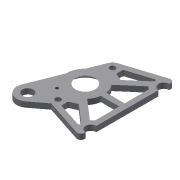
# Autodesk Inventor part: v2_tri_headplate_parameter_REF
Saved by Autodesk Inventor 2019 (Build 230136000, 136)
## iProperties
Created: 2017-06-27
Part Number: v2_tri_headplate_parameter_REF
Material: Generic
Document SubType Name: Modeling
Designer: richp
Density: 1 g/cm^3
Appearance: Default
headplate_aperture_diameter: 0.450 in
headplate_thickness: 0.124 in
ball_bearing_radius: 0.125 in
Author: richp
Autodesk Inventor part; units mm, degrees
sketch "Sketch1" plane through (0, 0, 0) normal (0, 1, 0) x (-1, 0, 0)
  circle A0 centre (0, 0) radius 5.715
  circle A1 centre (0, 0) radius 24.4983 construction
  line L0 (38.3553, 0) -> (-43.5095, 0) construction
  line L1 (0, -41.4931) -> (0, 53.8329) construction
  line L2 (-24.4983, 0) -> (-24.4983, -14.859)
  arc A2 (-24.4983, -24.384) -> (-24.4983, -18.034) centre (-24.4983, -21.209) ccw
  arc A3 (-24.4983, 24.384) -> (-24.4983, 18.034) centre (-24.4983, 21.209) ccw construction
  line L3 (-24.4983, 21.209) -> (-24.4983, 18.034) construction
  arc A4 (-24.4983, 14.859) -> (-21.3233, 15.7097) centre (-24.4983, 21.209) ccw construction
  arc A5 (-21.9753, -27.0363) -> (-20.631, -26.2455) centre (-24.4983, -21.209) ccw construction
  line L4 (-24.4983, 14.859) -> (-24.4983, 0)
  line L5 (-24.4983, -14.859) -> (-24.4983, -18.034)
  arc A6 (-22.4188, -15.2092) -> (-24.4983, -27.559) centre (-24.4983, -21.209) ccw construction
  arc A7 (-24.4983, -18.034) -> (-24.4983, -24.384) centre (-24.4983, -21.209) ccw construction
  line L6 (-24.4983, 21.209) -> (-24.4983, 24.384) construction
  arc A8 (-24.4983, 18.034) -> (-24.4983, 24.384) centre (-24.4983, 21.209) ccw
  line L7 (-24.4983, 24.384) -> (-24.4983, 25.0867)
  line L8 (-24.4983, -24.384) -> (-24.4983, -25.0929)
  line L9 (-24.4983, 18.034) -> (-24.4983, 14.859)
  line L10 (-24.4983, -18.034) -> (-24.4983, -24.384) construction
  line L11 (0, 0) -> (-8.1614, 7.0656) construction
  line L12 (0, 0) -> (-8.1614, -7.0656) construction
  line L13 (0, 0) -> (24.493, 0) construction
  arc A9 (9.9646, -4.1519) -> (9.9646, 4.1519) centre (0, 0) ccw construction
  line L14 (-5.7223, -9.1535) -> (-5.719, -9.1507) construction
  line L15 (-9.8786, -4.3527) -> (-22.4188, -15.2092) construction
  line L16 (-21.3233, 15.7097) -> (-21.3233, -15.7097)
  arc A10 (7.4735, -7.7897) -> (9.7402, -4.654) centre (0, 0) ccw construction
  line L17 (-5.719, -9.1507) -> (-18.2625, -20.01) construction
  arc A11 (-18.1902, -21.9377) -> (-18.2625, -20.01) centre (-24.4983, -21.209) ccw construction
  arc A12 (-18.2625, -20.01) -> (-19.6975, -17.0527) centre (-24.4983, -21.209) ccw construction
  line L18 (-8.1614, -7.0656) -> (-19.6975, -17.0527)
  arc A13 (-19.6975, -17.0527) -> (-21.3233, -15.7097) centre (-24.4983, -21.209) ccw
  arc A14 (-8.1614, 7.0656) -> (-8.1614, -7.0656) centre (0, 0) ccw
  line L19 (-19.6975, 17.0527) -> (-24.4983, 21.209) construction
  arc A15 (-21.3233, 15.7097) -> (-19.6975, 17.0527) centre (-24.4983, 21.209) ccw
  arc A16 (-21.3233, -15.7097) -> (-22.4188, -15.2092) centre (-24.4983, -21.209) ccw construction
  line L20 (-8.1614, 7.0656) -> (-18.5216, 16.0348)
  arc A17 (-8.1614, -7.0656) -> (6.5744, -8.562) centre (0, 0) ccw construction
  line L21 (-8.1614, -7.0656) -> (-19.6975, -17.0527) construction
  arc A18 (-21.3233, -15.7097) -> (-24.4983, -14.859) centre (-24.4983, -21.209) ccw construction
  line L22 (-19.6975, -17.0527) -> (-24.4983, -21.209) construction
  arc A19 (-19.6975, -17.0527) -> (-21.3233, -15.7097) centre (-24.4983, -21.209) ccw construction
  line L23 (-18.5216, 16.0348) -> (-19.6975, 17.0527)
  arc A20 (-19.6975, 17.0527) -> (-18.7927, 23.9963) centre (-24.4983, 21.209) ccw construction
  arc A21 (9.9646, 4.1519) -> (8.0122, 7.2344) centre (0, 0) ccw construction
  arc A22 (7.4735, 7.7897) -> (5.3975, 9.3487) centre (0, 0) ccw construction
  line L24 (0, 0) -> (5.3975, 9.3487) construction
  circle A23 centre (12.2491, 21.2162) radius 3.175
  arc A24 (15.4241, 26.7154) -> (12.0688, 27.5636) centre (12.2491, 21.2162) ccw
  arc A25 (17.9787, 18.4785) -> (18.1476, 18.8644) centre (12.2491, 21.2162) ccw construction
  arc A26 (12.0688, 27.5636) -> (8.7197, 26.4949) centre (12.2491, 21.2162) ccw
  arc A27 (-24.4983, -27.559) -> (-22.566, -27.2579) centre (-24.4983, -21.209) ccw construction
  arc A28 (-20.631, -26.2455) -> (-18.1902, -21.9377) centre (-24.4983, -21.209) ccw construction
  arc A29 (-20.631, -26.2455) -> (-19.6975, -17.0527) centre (-24.4983, -21.209) ccw construction
  arc A30 (6.5744, -8.562) -> (7.4735, -7.7897) centre (0, 0) ccw construction
  arc A31 (9.7402, -4.654) -> (9.9646, -4.1519) centre (0, 0) ccw construction
  arc A32 (6.7499, 18.0412) -> (7.1395, 17.446) centre (12.2491, 21.2162) ccw construction
  arc A33 (6.7484, 24.3886) -> (6.7499, 18.0412) centre (12.2491, 21.2162) ccw construction
  arc A34 (-0.7648, 10.7679) -> (-8.1614, 7.0656) centre (0, 0) ccw construction
  arc A35 (-18.7927, 23.9963) -> (-18.999, 24.384) centre (-24.4983, 21.209) ccw construction
  arc A36 (-18.999, 24.384) -> (-21.9753, 27.0363) centre (-24.4983, 21.209) ccw construction
  arc A37 (-21.9753, 27.0363) -> (-22.5177, 27.2422) centre (-24.4983, 21.209) ccw construction
  arc A38 (-24.4987, 27.559) -> (-24.4983, 14.859) centre (-24.4983, 21.209) ccw construction
  arc A39 (0, -11.8491) -> (3.716, -17.3312) centre (0, -15.8496) ccw construction
  circle A40 centre (0, 15.8496) radius 4.0005 construction
  line L25 (3.0165, -19.0856) -> (3.716, -17.3312) construction
  arc A41 (18.1476, 18.8644) -> (15.4241, 26.7154) centre (12.2491, 21.2162) ccw
  line L26 (3.0165, -19.0856) -> (1.2173, -19.6604) construction
  arc A42 (9.0741, 15.7169) -> (11.5389, 14.906) centre (12.2491, 21.2162) ccw construction
  arc A43 (5.3975, 9.3487) -> (2.2591, 10.556) centre (0, 0) ccw construction
  line L27 (9.0741, 15.7169) -> (22.677, 39.2777) construction
  line L28 (5.3975, 9.3487) -> (9.0741, 15.7169) construction
  arc A44 (11.5389, 14.906) -> (17.9787, 18.4785) centre (12.2491, 21.2162) ccw construction
  arc A45 (7.1395, 17.446) -> (9.0741, 15.7169) centre (12.2491, 21.2162) ccw construction
  arc A46 (2.2591, 10.556) -> (1.3866, 10.7056) centre (0, 0) ccw construction
  arc A47 (8.0122, 7.2344) -> (7.4735, 7.7897) centre (0, 0) ccw construction
  arc A48 (8.7197, 26.4949) -> (18.1476, 18.8644) centre (12.2491, 21.2162) ccw construction
  arc A49 (-22.5656, 27.2577) -> (-24.4983, 27.559) centre (-24.4983, 21.209) ccw construction
  arc A50 (-22.566, -27.2579) -> (-20.631, -26.2455) centre (-24.4983, -21.209) ccw construction
  arc A51 (3.716, -17.3312) -> (0, -11.8491) centre (0, -15.8496) ccw construction
  line L29 (0, -20.0493) -> (-21.848, -27.0285)
  arc A52 (1.2173, -19.6604) -> (3.716, -17.3312) centre (0, -15.8496) ccw
  line L30 (0, 19.8501) -> (-21.8325, 27.0173)
  arc A53 (-22.5177, 27.2422) -> (-22.5656, 27.2577) centre (-24.4983, 21.209) ccw construction
  line L31 (0, 19.8501) -> (8.3945, 26.2624)
  arc A54 (8.3945, 26.2624) -> (6.7484, 24.3886) centre (12.2491, 21.2162) ccw construction
  arc A55 (-21.8325, 27.0173) -> (-24.4983, 25.0867) centre (-22.4663, 25.0867) ccw
  arc A56 (-24.4983, -25.0929) -> (-21.848, -27.0285) centre (-22.4663, -25.0929) ccw
  line L32 (-21.8325, 27.0173) -> (-24.4983, 27.8924) construction
  line L33 (-24.4983, 24.384) -> (-24.4983, 27.8924) construction
  line L34 (-21.848, -27.0285) -> (-24.4983, -27.8751) construction
  line L35 (-24.4983, -25.0929) -> (-24.4983, -27.8751) construction
  line L36 (8.3945, 26.2624) -> (26.6603, 40.2149) construction
  line L37 (18.1476, 18.8644) -> (26.6603, 40.2149) construction
  line L38 (1.2173, -19.6604) -> (0, -20.0493)
  line L39 (3.716, -17.3312) -> (18.1476, 18.8644)
  arc A57 (18.1476, 18.8644) -> (8.3945, 26.2624) centre (12.2491, 21.2162) ccw
  dimension "headplate_aperture_diameter" = 11.43
  dimension "mount_diameter" = 48.9966
  dimension "d3" = 6.35
  dimension "d4" = 42.418
  dimension "d5" = 31.6992
  dimension "d7" = 3.175
  dimension "d8" = 3.175
  dimension "d10" = 5.08
  dimension "d11" = 3.175
  dimension "d12" = 3.175
  dimension "d16" = 3.175
  dimension "d33" = 120
  dimension "d34" = 6.35
  dimension "d36" = 3.175
  dimension "d46" = 8.001
  dimension "d75" = 2.032
  constraints: 143 point on circle, 76 end point, 57 centre point, 26 tangent, 16 point on line, 11 collinear, 10 vertical, 6 coincident, 4 symmetric about line, 3 parallel, 1 equal radius, 1 horizontal, 1 midpoint, 1 vertical alignment, 5 other
  measures "headplate_aperture_diameter" diameter of A0
  measures "mount_diameter" diameter of A1
  measures "d3" diameter of A2
  measures "d4" distance of L3.start A2.centre
  measures "d5" distance of point (0, -15.85) point (0, 15.85)
  measures "d7" radial gap between concentric circles of A3 A4
  measures "d8" radial gap between concentric circles of A2 A5
  measures "d10" radial gap between concentric circles of A0 A9
  measures "d11" distance between parallel lines of L12 L14
  measures "d12" distance between parallel lines of L12 L15
  measures "d16" distance between parallel lines of L4 L16
  measures "d33" angle of L0 L24
  measures "d34" diameter of A23
  measures "d36" radial gap between concentric circles of A23 A24
  measures "d46" diameter of A39
  measures "d75" radius of A55
ref_plane "Work Plane2" through (0, 1.524, 0) normal (0, 1, 0) x (1, 0, 0)
ref_plane "Work Plane4" through (0, 1.524, 0) normal (0, 1, 0) x (1, 0, 0)
extrude "Extrusion6" add sketch "Sketch1" against normal blind 3.1496
sketch "Sketch6" plane through (0, 0, 0) normal (0, 1, 0) x (1, 0, 0)
  point P0 (0, 0)
  point P1 (0, -15.8496)
  point P2 (0, 15.8496)
hole "Hole4" [suppressed]
chamfer "Chamfer2" [suppressed]
sketch "Sketch7" plane through (0, -3.1496, 0) normal (0, -1, 0) x (1, 0, 0)
  point P0 (0, 0)
  point P1 (0, 15.8496)
  point P2 (0, -15.8496)
hole "Hole5" at (0, -3.1496, -15.8496) at (0, -3.1496, 15.8496) direction (0, 1, 0) diameter 3.2766 depth 8.8646 tip angle 118 countersink diameter 5.715 countersink angle 82 clearance for "Flat Head Machine Screw (82)" size "#4" standard "Ansi Unified Screw Threads"
chamfer "Chamfer3" distance 3.1496 angle 45 1 edges at (5.715, -3.1496, 0)
ref_plane "Work Plane5" through (0, -3.1496, 0) normal (0, -1, 0) x (1, 0, 0)
sketch "Sketch8" plane through (0, -3.1496, 0) normal (0, -1, 0) x (1, 0, 0)
  point P0 (0, 0)
  point P1 (0, 0)
  point P2 (0, 0)
  constraints: 1 coincident
hole "Hole6" [suppressed]
sketch "Sketch9" plane through (0, 0, 0) normal (0, 1, 0) x (1, 0, 0)
  arc A0 (8.1614, -7.0656) -> (8.1614, 7.0656) centre (0, 0) ccw projected
  line L0 (19.6975, 17.0527) -> (8.1614, 7.0656) projected
  line L1 (8.1614, -7.0656) -> (19.6975, -17.0527) projected
  line L2 (10.795, 9.3456) -> (10.795, 0)
  line L3 (10.795, 0) -> (10.795, -9.3456)
  line L4 (8.1614, 7.0656) -> (19.6975, 17.0527) projected
  line L5 (10.795, 9.3456) -> (8.1614, 7.0656)
  line L6 (10.795, -9.3456) -> (8.1614, -7.0656)
  line L7 (19.6975, -17.0527) -> (8.1614, -7.0656) projected
  arc A1 (8.1614, -7.0656) -> (8.1614, 7.0656) centre (0, 0) ccw
  constraints: 8 end point, 4 point on circle, 3 point on line, 2 tangent, 2 vertical, 1 centre point, 1 coincident, 1 collinear
extrude "Extrusion7" [suppressed]
sketch "Sketch10" plane through (0, 0, 0) normal (0, 1, 0) x (1, 0, 0)
  line L0 (-3.716, 17.3312) -> (-18.1476, -18.8644) projected
  arc A0 (-9.9646, 4.1519) -> (-9.9646, -4.1519) centre (0, 0) ccw construction
  arc A1 (-7.4735, 7.7897) -> (-9.7402, 4.654) centre (0, 0) ccw construction
  line L1 (-18.1476, -18.8644) -> (-3.716, 17.3312) projected
  arc A2 (-8.4953, 6.6604) -> (-10.7874, -0.4044) centre (0, 0) ccw
  line L2 (-10.7874, -0.4044) -> (-7.5498, 7.7157)
  arc A3 (-7.5498, 7.7157) -> (-8.4953, 6.6604) centre (0, 0) ccw
  constraints: 6 point on circle, 2 centre point, 2 coincident, 2 end point, 2 point on line
extrude "Extrusion8" add sketch "Sketch10" against normal blind 3.1496
sketch "Sketch11" plane through (0, -3.1496, 0) normal (0, -1, 0) x (1, 0, 0)
  line L0 (24.4983, -18.034) -> (24.4983, 18.034) projected
  arc A0 (24.4983, 24.384) -> (24.4983, 18.034) centre (24.4983, 21.209) ccw projected
  line L1 (24.4983, 24.384) -> (24.4983, 25.0867) projected
  arc A1 (24.4983, 25.0867) -> (21.8325, 27.0173) centre (22.4663, 25.0867) ccw projected
  line L2 (21.8325, 27.0173) -> (0, 19.8501) projected
  line L3 (0, 19.8501) -> (-8.3945, 26.2624) projected
  arc A2 (-8.3945, 26.2624) -> (-18.1476, 18.8644) centre (-12.2491, 21.2162) ccw projected
  line L4 (-18.1476, 18.8644) -> (-10.7874, 0.4044) projected
  arc A3 (-3.716, -17.3312) -> (-1.2173, -19.6604) centre (0, -15.8496) ccw projected
  line L5 (-1.2173, -19.6604) -> (21.848, -27.0285) projected
  arc A4 (21.848, -27.0285) -> (24.4983, -25.0929) centre (22.4663, -25.0929) ccw projected
  line L6 (24.4983, -25.0929) -> (24.4983, -24.384) projected
  arc A5 (24.4983, -18.034) -> (24.4983, -24.384) centre (24.4983, -21.209) ccw projected
  circle A6 centre (-12.2491, 21.2162) radius 3.175 projected
  arc A7 (21.3233, -15.7097) -> (19.6975, -17.0527) centre (24.4983, -21.209) ccw projected
  line L7 (19.6975, -17.0527) -> (8.1614, -7.0656) projected
  line L8 (8.1614, 7.0656) -> (19.6975, 17.0527) projected
  arc A8 (19.6975, 17.0527) -> (21.3233, 15.7097) centre (24.4983, 21.209) ccw projected
  line L9 (21.3233, 15.7097) -> (21.3233, -15.7097) projected
  circle A9 centre (0, 15.8496) radius 2.8575 projected
  circle A10 centre (0, -15.8496) radius 2.8575 projected
  line L10 (4.5527, -18.1705) -> (17.9673, -22.4558)
  line L11 (-1.2173, -19.6604) -> (21.848, -27.0285) projected
  line L12 (8.7283, -12.4421) -> (18.7283, -21.0995)
  line L13 (19.6975, -17.0527) -> (8.1614, -7.0656) projected
  arc A11 (17.9673, -22.4558) -> (18.7283, -21.0995) centre (18.2088, -21.6996) ccw
  line L14 (4.0005, -17.4144) -> (4.0005, -14.5718)
  arc A12 (-3.716, -17.3312) -> (-1.2173, -19.6604) centre (0, -15.8496) ccw projected
  circle A13 centre (0, -15.8496) radius 4.0005 construction
  arc A14 (-6.5744, -8.562) -> (8.1614, -7.0656) centre (0, 0) ccw construction
  line L15 (0, -15.8496) -> (4.0005, -14.0576) construction
  line L16 (4.0005, -14.0576) -> (12.065, -10.4451) construction
  line L17 (4.4698, -13.8474) -> (7.8842, -12.3179)
  arc A15 (4.0005, -17.4144) -> (4.5527, -18.1705) centre (4.7942, -17.4144) ccw
  arc A16 (4.4698, -13.8474) -> (4.0005, -14.5718) centre (4.7942, -14.5718) ccw
  arc A17 (8.7283, -12.4421) -> (7.8842, -12.3179) centre (8.2087, -13.0422) ccw
  line L18 (-30.1541, 0) -> (34.1819, 0) projected
  line L19 (4.5527, 18.1705) -> (17.9673, 22.4558)
  line L20 (8.7283, 12.4421) -> (18.7283, 21.0995)
  arc A18 (18.7283, 21.0995) -> (17.9673, 22.4558) centre (18.2088, 21.6996) ccw
  line L21 (4.0005, 17.4144) -> (4.0005, 14.5718)
  line L22 (4.4698, 13.8474) -> (7.8842, 12.3179)
  arc A19 (4.5527, 18.1705) -> (4.0005, 17.4144) centre (4.7942, 17.4144) ccw
  arc A20 (4.0005, 14.5718) -> (4.4698, 13.8474) centre (4.7942, 14.5718) ccw
  arc A21 (7.8842, 12.3179) -> (8.7283, 12.4421) centre (8.2087, 13.0422) ccw
  arc A22 (8.1614, -7.0656) -> (8.1614, 7.0656) centre (0, 0) ccw projected
  arc A23 (-10.7874, 0.4044) -> (-7.5498, -7.7157) centre (0, 0) ccw projected
  line L23 (-7.5498, -7.7157) -> (-3.716, -17.3312) projected
  point P0 (8.3458, -12.1111)
  point P1 (4.0005, 14.0576)
  dimension "d98" = 3.175
  dimension "d99" = 3.6938
  dimension "d100" = 0.7937
  dimension "d101" = 0.7937
  dimension "d102" = 0.7937
  constraints: 20 end point, 16 point on circle, 13 symmetric about line, 8 centre point, 8 point on line, 8 tangent, 2 parallel, 2 vertical, 1 coincident, 1 equal radius, 7 other
  measures "d98" distance between parallel lines of L5 L10
  measures "d99" distance between parallel lines of L7 L12
  measures "d100" radius of A11
  measures "d101" radius of A15
  measures "d102" radius of A16
extrude "Extrusion9" cut sketch "Sketch11" against normal blind 3.1496 contours A15 L14 A16 L17 A17 L12 A11 L10 | L19 A18 L20 A21 L22 A20 L21 A19
sketch "Sketch17" plane through (0, -3.1496, 0) normal (0, -1, 0) x (1, 0, 0)
  circle A0 centre (0, 0) radius 8.75 construction
  circle A1 centre (0, 0) radius 9 construction
  dimension "d123" = 18
  dimension "d124" = 17.5
  constraints: 2 centre point, 2 coincident
  measures "d123" diameter of A1
  measures "d124" diameter of A0
chamfer "Chamfer4" [suppressed]
sketch "Sketch18" plane through (0, -3.1496, 0) normal (0, -1, 0) x (1, 0, 0)
  circle A0 centre (0, 0) radius 8.8646 construction
  circle A1 centre (-12.2491, 21.2162) radius 3.175 projected
  circle A2 centre (-12.2491, 21.2162) radius 3.175 construction
  line L0 (-12.2491, 21.2162) -> (-4.4323, 7.677) construction
  circle A3 centre (0, 0) radius 5.715 construction
  line L1 (-2.8575, 4.9493) -> (0, 0) construction
  line L2 (-4.4323, 7.677) -> (-2.8575, 4.9493) construction
  arc A4 (-7.917, 3.9878) -> (0.505, 8.8502) centre (0, 0) ccw
  line L3 (-9.2794, 9.2143) -> (-8.003, 7.0035)
  line L4 (-8.1172, 13.5515) -> (-7.8973, 13.6785)
  line L5 (-3.3402, 12.6433) -> (-2.0638, 10.4325)
  line L6 (-7.6773, 13.8055) -> (-7.8973, 13.6785)
  arc A5 (-4.4323, 7.677) -> (-7.0569, 5.3649) centre (0, 0) ccw construction
  arc A6 (-1.1177, 8.7939) -> (-4.4323, 7.677) centre (0, 0) ccw construction
  arc A7 (-8.1172, 13.5515) -> (-9.2794, 9.2143) centre (-6.5297, 10.8018) ccw
  arc A8 (-3.3402, 12.6433) -> (-7.6773, 13.8055) centre (-6.0898, 11.0558) ccw
  arc A9 (-2.0638, 10.4325) -> (0.505, 8.8502) centre (0.6859, 12.02) ccw
  arc A10 (-7.917, 3.9878) -> (-8.003, 7.0035) centre (-10.7526, 5.416) ccw
  point P0 (-10.8669, 11.964)
  point P1 (-4.9277, 15.393)
  dimension "d128" = 7.62
  dimension "d129" = 3.429
  dimension "d142" = 3.175
  constraints: 16 point on circle, 14 end point, 9 point on line, 8 tangent, 7 centre point, 3 equal radius, 2 symmetric about line, 1 coincident, 1 parallel, 1 perpendicular, 5 other
  measures "d128" distance of point (-10.867, 11.964) A5.end
  measures "d129" distance of point (-10.867, 11.964) L4.end
  measures "d142" radius of A10
extrude "Extrusion10" cut sketch "Sketch18" against normal blind 1.5748 contours A10 L3 A7 L4 L6 A8 L5 A9 A4
sketch "Sketch19" plane through (0, -1.5748, 0) normal (0, -1, 0) x (1, 0, 0)
  circle A0 centre (0, 0) radius 7.2898 projected
  line L0 (-8.1172, 13.5515) -> (-7.6773, 13.8055) projected
  arc A1 (-8.1172, 13.5515) -> (-9.2794, 9.2143) centre (-6.5297, 10.8018) ccw projected
  line L1 (-8.003, 7.0035) -> (-9.2794, 9.2143) projected
  arc A2 (-7.917, 3.9878) -> (-8.003, 7.0035) centre (-10.7526, 5.416) ccw projected
  arc A3 (-7.917, 3.9878) -> (0.505, 8.8502) centre (0, 0) ccw projected
  arc A4 (-2.0638, 10.4325) -> (0.505, 8.8502) centre (0.6859, 12.02) ccw projected
  line L2 (-3.3402, 12.6433) -> (-2.0638, 10.4325) projected
  arc A5 (-3.3402, 12.6433) -> (-7.6773, 13.8055) centre (-6.0898, 11.0558) ccw projected
  point P0 (-6.0325, 10.4486)
  dimension "d133" = 12.065
  dimension "d134" = 3.429
  measures "d133" distance of point (0, 0) point (-6.032, 10.449)
  measures "d134" distance from line of L2 point (-6.032, 10.449)
hole "Hole9" at (-6.0325, -1.5748, 10.4486) direction (0, 1, 0) diameter 1.7018 depth 6.6294 tip angle 118
sketch "Sketch20" plane through (0, 0, 0) normal (0, 1, 0) x (1, 0, 0)
  line L0 (-38.3553, 0) -> (43.5095, 0) construction
  line L1 (23.2205, -1.5875) -> (10.0043, -1.5875)
  line L2 (10.0043, -1.5875) -> (10.0043, 1.5875)
  line L3 (10.0043, 1.5875) -> (23.2205, 1.5875)
  line L4 (23.2205, 1.5875) -> (23.2205, -1.5875)
  line L5 (23.2205, -1.5875) -> (10.0043, 1.5875) construction
  line L6 (10.0043, -1.5875) -> (23.2205, 1.5875) construction
  arc A0 (8.1614, -7.0656) -> (8.1614, 7.0656) centre (0, 0) ccw projected
  line L7 (21.3233, -15.7097) -> (21.3233, 15.7097) projected
  point P0 (16.6124, 0)
  dimension "d143" = 3.175
  dimension "d144" = 1.8972
  dimension "d145" = 13.2162
  constraints: 12 end point, 2 midpoint, 2 parallel, 1 horizontal, 1 perpendicular, 1 point on line
  measures "d143" distance between parallel lines of L1 L3
  measures "d144" distance between parallel lines of L7 L4
  measures "d145" distance between parallel lines of L2 L4
extrude "Extrusion11" add sketch "Sketch20" against normal blind 3.1496
equation "\"d4\" = bearing_edge_distance"
equation "\"d7\" = ball_bearing_radius"
equation "\"d8\" = ball_bearing_radius"
equation "\"d36\" = d7"
equation "\"bearing_edge_distance\" = 42.418"
equation "\"headplate_thickness\" = 3.1496"
equation "\"center_thread_major_diameter\" = 18"
equation "\"center_thread_minor_diameter\" = 17.5"
equation "\"ball_bearing_radius\" = 3.175"
body "Solid1"
